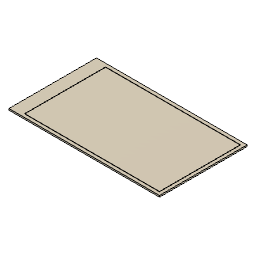
Spectra6_4in (Autodesk Fusion 360 archive; units mm, degrees)
design "epd3.97"
part number: 2026-03-13-14-33-30-724
Autodesk Fusion 360 part; units mm, degrees
sketch "Sketch1" plane through (0, 0, 0) normal (0, 1, 0) x (1, 0, 0)
  line L0 (48.31, 28.12) -> (-48.31, 28.12)
  line L1 (-48.31, 28.12) -> (-48.31, -28.12)
  line L2 (-48.31, -28.12) -> (48.31, -28.12)
  line L3 (48.31, -28.12) -> (48.31, 28.12)
  line L4 (48.31, 28.12) -> (-48.31, -28.12) construction
  line L5 (-48.31, 28.12) -> (48.31, -28.12) construction
  line L6 (46.11, 25.92) -> (-40.29, 25.92)
  line L7 (-40.29, 25.92) -> (-40.29, -25.92)
  line L8 (-40.29, -25.92) -> (46.11, -25.92)
  line L9 (46.11, -25.92) -> (46.11, 25.92)
  line L10 (46.11, 25.92) -> (-40.29, -25.92) construction
  line L11 (-40.29, 25.92) -> (46.11, -25.92) construction
  point P0 (4.4468, -0.9221)
  dimension "d193" = 96.62
  dimension "d194" = 56.24
  dimension "d195" = 86.4
  dimension "d196" = 51.84
  dimension "d197" = 2.2
  dimension "d198" = 2.2
  constraint horizontal L0
  constraint perpendicular L0 L1
  constraint parallel L0 L2
  constraint parallel L1 L3
  constraint coincident L4 origin
  constraint coincident L5 origin
  constraint horizontal L6
  constraint perpendicular L6 L7
  constraint parallel L6 L8
  constraint parallel L7 L9
  constraint coincident L11 P0
  measures "d193" distance of L1.end L2.end
  measures "d194" distance of L0.end L1.end
  measures "d195" distance of L7.end L8.end
  measures "d196" distance of L6.end L7.end
  measures "d197" distance of L3 L9
  measures "d198" distance of L0 L6
extrude "Extrude1" add sketch "Sketch1" against normal blind 1 contours L0 L1 L2 L3 | L6 L7 L8 L9
extrude "Extrude2" cut sketch "Sketch1" against normal blind 0.1 contours L6 L7 L8 L9
sketch "Sketch3" plane through (0, -1, 0) normal (0, -1, 0) x (1, 0, 0)
  line L0 (48.31, -28.12) -> (48.31, 28.12)
  line L1 (48.31, 28.12) -> (-48.31, 28.12)
  line L2 (-48.31, 28.12) -> (-48.31, -28.12)
  line L3 (-48.31, -28.12) -> (48.31, -28.12)
  line L4 (-14.65, -28.21) -> (-11.65, -28.21)
  line L5 (-11.65, -28.21) -> (-11.65, -15.71)
  line L6 (-11.65, -15.71) -> (-14.65, -15.71)
  line L7 (-14.65, -15.71) -> (-14.65, -28.21)
  line L8 (-14.65, -28.21) -> (-11.65, -15.71) construction
  line L9 (-11.65, -28.21) -> (-14.65, -15.71) construction
  line L10 (-48.31, 28.12) -> (48.31, 28.12)
  line L11 (-48.31, -28.12) -> (-48.31, 28.12)
  point P0 (-13.15, -21.96)
  dimension "d1" = 3
  dimension "d2" = 12.5
  dimension "d3" = 43.83
  dimension "d4" = 33.66
  constraint horizontal L4
  constraint perpendicular L4 L5
  constraint parallel L4 L6
  constraint parallel L5 L7
  constraint coincident L8 P0
  constraint coincident L9 P0
  measures "d1" distance of L5.end L6.end
  measures "d2" distance of L4.end L5.end
  measures "d3" distance of L6 L10
  measures "d4" distance of L7 L11
extrude "Extrude3" add sketch "Sketch3" along normal blind 0.5 contours L3 L5 L6 L7
